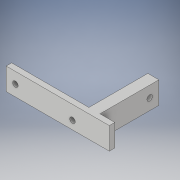
# Autodesk Inventor part: thumper-bumper-solenoid-interface-v2
Saved by Autodesk Inventor 2017 (Build 210142000, 142)
## iProperties
Created: 2017-02-22
Part Number: thumper-bumper-solenoid-interface-v2
Material: Generic
Document SubType Name: Modeling
Designer: John
Density: 1 g/cm^3
Appearance: Default
Author: John
Autodesk Inventor part; units mm, degrees
ref_plane "YZ Plane" through (0, 0, 0) normal (1, 0, 0) x (0, 1, 0)
ref_plane "XZ Plane" through (0, 0, 0) normal (0, 1, 0) x (-1, 0, 0)
ref_plane "XY Plane" through (0, 0, 0) normal (0, 0, 1) x (1, 0, 0)
sketch "Sketch3" plane through (0, 0, 0) normal (0, 0, 1) x (1, 0, 0)
  line L0 (0, 0) -> (56, 0)
  line L1 (56, 0) -> (56, 12)
  line L2 (56, 12) -> (0, 12)
  line L3 (0, 12) -> (0, 0)
  circle A0 centre (36, 4.5) radius 1.5
  circle A1 centre (5, 6) radius 1.5
  dimension "d0" = 56
  dimension "d2" = 3
  dimension "d3" = 4.5
  dimension "d4" = 12
  dimension "d8" = 20
  dimension "d17" = 3
  dimension "d18" = 5
  constraints: 8 end point, 2 centre point, 2 parallel, 1 horizontal, 1 perpendicular
  measures "d0" distance of L2.end L1.end
  measures "d2" diameter of A0
  measures "d3" distance from line of L0 A0.centre
  measures "d4" distance of L0.end L1.end
  measures "d8" distance from line of L1 A0.centre
  measures "d17" diameter of A1
  measures "d18" distance from line of A1.centre L3
extrude "Extrusion1" add sketch "Sketch3" along normal blind 3
sketch "Sketch4" plane through (0, 0, 3) normal (0, 0, 1) x (1, 0, 0)
  line L0 (56, 12) -> (0, 12) projected
  line L1 (41.9, 0) -> (47.9, 0)
  line L2 (47.9, 0) -> (47.9, 12)
  line L3 (47.9, 12) -> (41.9, 12)
  line L4 (41.9, 12) -> (41.9, 0)
  circle A0 centre (36, 4.5) radius 1.5 projected
  point P0 (0, 0)
  dimension "d9" = 6
  dimension "d10" = 5.9
  constraints: 8 end point, 2 parallel, 1 horizontal, 1 perpendicular, 1 point on line
  measures "d9" distance of L3.end L2.end
  measures "d10" distance from line of L4 A0.centre
extrude "Extrusion2" add sketch "Sketch4" against normal blind 35 contours L2 L1 L4 L0
sketch "Sketch5" plane through (47.9, 0, 0) normal (1, 0, 0) x (0, 0, -1)
  line L0 (32, 0) -> (32, 12) construction
  line L1 (0, 6) -> (0, 3) construction
  line L2 (32, 6) -> (0, 6) construction
  circle A0 centre (27, 6) radius 1.5
  point P0 (0, 0)
  dimension "d13" = 3
  dimension "d14" = 5
  constraints: 2 end point, 1 centre point, 1 horizontal, 1 midpoint, 1 point on line
  measures "d13" diameter of A0
  measures "d14" distance from line of L0 A0.centre
extrude "Extrusion3" cut sketch "Sketch5" against normal through all
body "Solid1"
